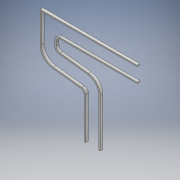
# Autodesk Inventor part: rail
Saved by Autodesk Inventor 2017 (Build 210142000, 142)
## iProperties
Part Number: rail
Material: Générique
Document SubType Name: Modeling
Designer: Thomas
Density: 1 g/cm^3
Appearance: Par défaut
Author: Thomas
Autodesk Inventor part; units mm, degrees
ref_plane "YZ Plane" through (0, 0, 0) normal (1, 0, 0) x (0, 1, 0)
ref_plane "XZ Plane" through (0, 0, 0) normal (0, 1, 0) x (-1, 0, 0)
ref_plane "XY Plane" through (0, 0, 0) normal (0, 0, 1) x (1, 0, 0)
sketch "Esquisse1" plane through (0, 0, 0) normal (0, 1, 0) x (-1, 0, 0)
  line L0 (0, 0) -> (300, 0) construction
  line L1 (300, 0) -> (300, -300) construction
  line L2 (0, -300) -> (0, 0) construction
  line L3 (158.1666, -300) -> (158.1666, -290) construction
  line L4 (158.1666, -290) -> (158.1666, -210) construction
  line L5 (158.1666, -210) -> (258.1666, -210) construction
  line L6 (258.1666, -210) -> (258.1666, -159) construction
  line L7 (202.1666, -154) -> (102.1666, -154) construction
  line L8 (102.1666, -300) -> (102.1666, -154) construction
  line L9 (202.1666, -136) -> (102.1666, -136) construction
  line L10 (215.9662, -80) -> (258.1666, -80) construction
  line L11 (258.1666, -80) -> (258.1666, -159) construction
  line L12 (215.9662, -80) -> (102.1666, -80) construction
  line L13 (202.1666, -136) -> (202.1666, -154) construction
  line L14 (102.1666, -136) -> (18.7834, -136) construction
  line L15 (18.7834, -136) -> (18.7834, -80) construction
  line L16 (18.7834, -80) -> (102.1666, -80) construction
  line L17 (300, -300) -> (158.1666, -300) construction
  line L18 (102.1666, -300) -> (0, -300)
  line L19 (248.1666, -159) -> (248.1666, -188.7363)
  line L20 (148.1666, -203.3121) -> (148.1666, -290)
  line L21 (148.1666, -290) -> (148.1666, -300)
  line L22 (112.1666, -300) -> (112.1666, -169.4638)
  line L23 (212.1666, -152.1462) -> (212.1666, -126)
  line L24 (212.1666, -126) -> (102.1666, -126)
  line L25 (102.1666, -126) -> (28.7834, -126)
  line L26 (28.7834, -90) -> (102.1666, -90)
  line L27 (102.1666, -90) -> (215.9662, -90)
  line L28 (215.9662, -90) -> (248.1666, -90)
  line L29 (248.1666, -90) -> (248.1666, -159)
  line L30 (148.1666, -300) -> (112.1666, -300) construction
  line L31 (28.7834, -123) -> (102.1666, -123)
  line L32 (102.1666, -123) -> (215.1666, -123)
  line L33 (215.1666, -123) -> (215.1666, -155.574)
  line L34 (115.1666, -170.9458) -> (115.1666, -297)
  line L35 (145.1666, -297) -> (145.1666, -290)
  line L36 (145.1666, -290) -> (145.1666, -203.3246)
  line L37 (245.1666, -185.6192) -> (245.1666, -159)
  line L38 (245.1666, -159) -> (245.1666, -93)
  line L39 (245.1666, -93) -> (215.9662, -93)
  line L40 (215.9662, -93) -> (102.1666, -93)
  line L41 (102.1666, -93) -> (28.7834, -93)
  line L42 (145.1666, -297) -> (145.1666, -300)
  line L43 (115.1666, -297) -> (115.1666, -300)
  line L44 (28.7834, -90) -> (28.7834, -93)
  line L45 (28.7834, -123) -> (28.7834, -126)
  line L46 (148.1666, -300) -> (145.1666, -300)
  line L47 (115.1666, -300) -> (112.1666, -300)
  line L48 (145.1666, -197) -> (145.1666, -203.3246)
  line L49 (148.1666, -203.3121) -> (148.1666, -200.1623)
  line L50 (112.1666, -164) -> (112.1666, -169.4638)
  line L51 (115.1666, -167) -> (115.1666, -170.9458)
  line L52 (148.1666, -200.1623) -> (245.1666, -189.0791)
  line L53 (115.1666, -167) -> (215.1666, -155.574)
  line L54 (245.1666, -189.0791) -> (248.1666, -188.7363)
  line L55 (145.1666, -197) -> (245.1666, -185.6192)
  line L56 (112.1666, -164) -> (212.1666, -152.1462)
  point P0 (212.1666, -155.9168)
  point P1 (115.1666, -164)
  dimension "d0" = 300
  dimension "d1" = 300
  dimension "d2" = 100
  dimension "d5" = 100
  dimension "d6" = 130
  dimension "d7" = 56
  dimension "d9" = 146
  dimension "d10" = 90
  dimension "d11" = 10
  dimension "d12" = 3
  constraints: 114 end point, 13 perpendicular, 5 point on line, 4 horizontal, 4 parallel, 4 vertical, 3 collinear, 8 other
  measures "d0" distance of L1.end L2.start
  measures "d1" distance of L0.end L1.end
  measures "d2" distance of L4.end L5.end
  measures "d5" distance of L7.start L7.end
  measures "d6" distance between parallel lines of L5 L10
  measures "d7" distance between parallel lines of L9 L12
  measures "d9" distance of L8.start L7.end
  measures "d10" distance between parallel lines of L17 L5
  measures "d11" distance between parallel lines of L6 L19
  measures "d12" distance between parallel lines of L29 L38
extrude "Extrusion1" add sketch "Esquisse1" along normal blind 6
fillet "Congé7" radius 30 2 edges at (-115.1666, 3, -167) (-112.1666, 3, -164)
fillet "Congé9" radius 10 2 edges at (-215.1666, 3, -123) (-212.1666, 3, -126)
fillet "Congé10" radius 10 2 edges at (-145.1666, 3, -197) (-148.1666, 3, -200.1623)
fillet "Congé11" radius 30 2 edges at (-245.1666, 3, -185.6192) (-248.1666, 3, -188.7363)
fillet "Congé12" radius 10 2 edges at (-215.1666, 3, -155.574) (-212.1666, 3, -152.1462)
